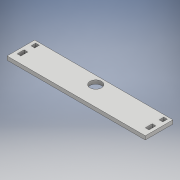
# Autodesk Inventor part: back
Saved by Autodesk Inventor 2018.3 (Build 223284000, 284)
## iProperties
Created: 2018-05-24
Part Number: back
Material: Generic
Document SubType Name: Modeling
Designer: mzhang
Density: 1 g/cm^3
Appearance: Default
Author: mzhang
Autodesk Inventor part; units mm, degrees
ref_plane "YZ Plane" through (0, 0, 0) normal (1, 0, 0) x (0, 1, 0)
ref_plane "XZ Plane" through (0, 0, 0) normal (0, 1, 0) x (-1, 0, 0)
ref_plane "XY Plane" through (0, 0, 0) normal (0, 0, 1) x (1, 0, 0)
sketch "Sketch1" plane through (0, 0, 0) normal (0, 0, 1) x (1, 0, 0)
  line L0 (0, 0) -> (54, 0)
  line L1 (54, 10) -> (52, 10)
  line L2 (0, 10) -> (0, 0)
  line L3 (0, 10) -> (-1.5875, 10)
  line L4 (-1.5875, 10) -> (-1.5875, 8)
  line L5 (-1.5875, 8) -> (0, 8)
  line L6 (0, 8) -> (0, 10)
  line L7 (0, 5) -> (-1.5875, 5)
  line L8 (-1.5875, 5) -> (-1.5875, 2)
  line L9 (-1.5875, 2) -> (0, 2)
  line L10 (0, 2) -> (0, 5)
  line L11 (27, 10) -> (27, -11.346)
  line L12 (54, 10) -> (55.5875, 10)
  line L13 (55.5875, 10) -> (55.5875, 8)
  line L14 (55.5875, 8) -> (54, 8)
  line L15 (54, 5) -> (55.5875, 5)
  line L16 (55.5875, 5) -> (55.5875, 2)
  line L17 (55.5875, 2) -> (54, 2)
  line L18 (57, -1) -> (-3, -1)
  line L19 (-3, -1) -> (-3, 11)
  line L20 (-3, 11) -> (57, 11)
  line L21 (57, 11) -> (57, -1)
  line L22 (57, -1) -> (27, 5) construction
  line L23 (-1.5875, 10.7175) -> (-3, 11) construction
  line L24 (-3, -1) -> (-1.5875, -0.7175) construction
  line L25 (27, 5) -> (57, 11) construction
  line L26 (54, 2) -> (54, 5)
  line L27 (54, 8) -> (54, 10)
  dimension "d0" = 54
  dimension "d1" = 10
  dimension "d2" = 2
  dimension "d3" = 1.5875
  dimension "d4" = 3
  dimension "d5" = 1.5875
  dimension "d6" = 3
  dimension "d7" = 60
  dimension "d8" = 12
  constraints: 56 end point, 9 parallel, 7 symmetric about line, 5 perpendicular, 4 horizontal, 4 point on line, 1 midpoint, 1 vertical
  measures "d0" distance of L2.start L1.start
  measures "d1" distance of L1.start L0.end
  measures "d2" distance of L4.end L3.end
  measures "d3" distance of L9.end L8.end
  measures "d4" distance of L8.end L7.end
  measures "d5" distance of L2.start L3.end
  measures "d6" distance between parallel lines of L7 L5
  measures "d7" distance of L19.end L20.end
  measures "d8" distance of L18.end L19.end
extrude "Extrusion1" add sketch "Sketch1" along normal blind 1.5875
sketch "Sketch2" plane through (0, 0, 1.5875) normal (0, 0, 1) x (1, 0, 0)
  circle A0 centre (27, 7.4899) radius 2.5
  point P0 (0, 0)
  dimension "d11" = 5
  constraints: 1 centre point
  measures "d11" diameter of A0
extrude "Extrusion2" cut sketch "Sketch2" against normal up to surface (1.5875 mm away)
body "Solid1"
